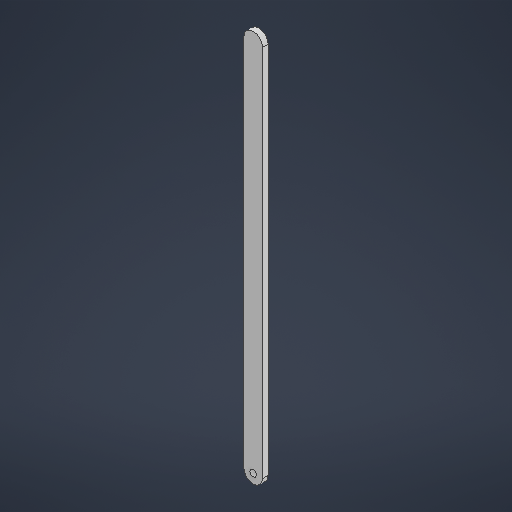
# Autodesk Inventor part: RedKangoroo_005_pata
Saved by Autodesk Inventor 2026.3 (Build 303398000, 398)
## iProperties
Created: 2026-05-22
Part Number: RedKangoroo_005_pata
Material: Generic
Document SubType Name: Modeling
Designer: ADMIN
Density: 1 g/cm^3
Appearance: Default
Author: ADMIN
Autodesk Inventor part; units mm, degrees
ref_plane "YZ Plane" through (0, 0, 0) normal (1, 0, 0) x (0, 1, 0)
ref_plane "XZ Plane" through (0, 0, 0) normal (0, 1, 0) x (-1, 0, 0)
ref_plane "XY Plane" through (0, 0, 0) normal (0, 0, 1) x (1, 0, 0)
sketch "Sketch1" plane through (0, 0, 0) normal (0, 0, 1) x (1, 0, 0)
  line L0 (0, 0) -> (0, 200.51) construction
  circle A0 centre (0, 0) radius 1.75
  line L1 (0, 0) -> (0, 200.51) construction
  line L2 (5, 0) -> (5, 200.51)
  line L3 (-5, 200.51) -> (-5, 0)
  arc A1 (-5, 0) -> (5, 0) centre (0, 0) ccw
  arc A2 (5, 200.51) -> (-5, 200.51) centre (0, 200.51) ccw
  point P0 (0, 100.255)
  point P1 (0, 100.255)
  dimension "d0" = 200.51
  dimension "d2" = 3.5
  dimension "d6" = 10
  constraints: 12 end point, 4 point on circle, 4 tangent, 3 centre point, 2 equal length, 2 midpoint, 1 coincident, 1 vertical
  measures "d0" distance of L0.start L0.end
  measures "d2" diameter of A0
  measures "d6" diameter of A2
extrude "Extrusion2" add sketch "Sketch1" along normal blind 3
body "Solid2"
